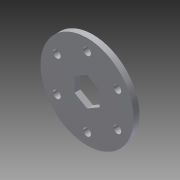
# Autodesk Inventor part: Hex Shaft Connector (Lexan)
Saved by Autodesk Inventor 2014 (Build 180170000, 170)
## iProperties
Created: 2014-02-11
Part Number: Hex Shaft Connector (Lexan)
Material: Aluminum 6061
Document SubType Name: Modeling
Designer: Michael
Density: 2.71 g/cm^3
Appearance: Aluminum - Flat
Author: Michael
Autodesk Inventor part; units mm, degrees
ref_plane "YZ Plane" through (0, 0, 0) normal (1, 0, 0) x (0, 1, 0)
ref_plane "XZ Plane" through (0, 0, 0) normal (0, 1, 0) x (-1, 0, 0)
ref_plane "XY Plane" through (0, 0, 0) normal (0, 0, 1) x (1, 0, 0)
sketch "Sketch1" plane through (0, 0, 0) normal (0, 0, 1) x (1, 0, 0)
  circle A0 centre (0, 0) radius 25.4
  circle A1 centre (0, 19.05) radius 2.0828
  line L0 (0, 0) -> (0, 19.05) construction
  circle A2 centre (-16.4978, 9.525) radius 2.0828
  circle A3 centre (-16.4978, -9.525) radius 2.0828
  circle A4 centre (0, -19.05) radius 2.0828
  circle A5 centre (16.4978, -9.525) radius 2.0828
  circle A6 centre (16.4978, 9.525) radius 2.0828
  line L1 (6.858, -3.9595) -> (0, -7.9189)
  line L2 (0, -7.9189) -> (-6.858, -3.9595)
  line L3 (-6.858, -3.9595) -> (-6.858, 3.9595)
  line L4 (-6.858, 3.9595) -> (0, 7.9189)
  line L5 (0, 7.9189) -> (6.858, 3.9595)
  line L6 (6.858, 3.9595) -> (6.858, -3.9595)
  dimension "d0" = 50.8
  dimension "d2" = 4.1656
  dimension "d3" = 19.05
  dimension "d6" = 360
  dimension "d10" = 13.716
  constraints: 14 end point, 7 centre point, 3 coincident, 2 vertical, 26 other
  measures "d0" diameter of A0
  measures "d2" diameter of A1
  measures "d3" distance of L0.end point (0, 0)
  measures "d10" distance between parallel lines of L2 L5
extrude "Extrusion1" add sketch "Sketch1" along normal blind 3.175
body "Solid1"
